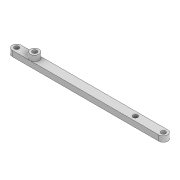
# Autodesk Inventor part: Part_5
Saved by Autodesk Inventor 2022 (Build 260153000, 153)
## iProperties
Created: 2022-04-21
Part Number: Part_5
Material: Generic
Document SubType Name: Modeling
Designer: dell
Density: 1 g/cm^3
Appearance: Default
Author: dell
Autodesk Inventor part; units mm, degrees
ref_plane "YZ Plane" through (0, 0, 0) normal (1, 0, 0) x (0, 1, 0)
ref_plane "XZ Plane" through (0, 0, 0) normal (0, 1, 0) x (-1, 0, 0)
ref_plane "XY Plane" through (0, 0, 0) normal (0, 0, 1) x (1, 0, 0)
sketch "Sketch1" plane through (0, 0, 0) normal (0, 1, 0) x (-1, 0, 0)
  line L0 (0, 0) -> (-132.537, 0) construction
  line L1 (0, 4) -> (-132.537, 4)
  line L2 (-132.537, -4) -> (0, -4)
  arc A0 (0, -4) -> (0, 4) centre (0, 0) ccw
  arc A1 (-132.537, 4) -> (-132.537, -4) centre (-132.537, 0) ccw
  circle A2 centre (0, 0) radius 2.1
  circle A3 centre (-16.286, 0) radius 2.1
  circle A4 centre (-132.537, 0) radius 2.1
  circle A5 centre (-107.252, 0) radius 2.1
  point P0 (-66.2685, 0)
  point P1 (-52.7225, 0)
  dimension "d0" = 132.537
  dimension "d1" = 8
  dimension "d2" = 4.2
  dimension "d8" = 4.2
  dimension "d9" = 16.286
  dimension "d10" = 4.2
  dimension "d28" = 4.2
  dimension "d29" = 107.252
  constraints: 8 end point, 6 centre point, 4 point on circle, 4 tangent, 2 coincident, 2 point on line, 1 horizontal, 1 midpoint, 1 parallel
  measures "d0" distance of L0.end L0.start
  measures "d1" distance between parallel lines of L1 L2
  measures "d2" diameter of A2
  measures "d8" diameter of A3
  measures "d9" distance of L0.start A3.centre
  measures "d10" diameter of A4
  measures "d28" diameter of A5
  measures "d29" distance of L0.start A5.centre
extrude "Extrusion1" add sketch "Sketch1" along normal blind 5
sketch "Sketch4" plane through (0, 5, 0) normal (0, 1, 0) x (1, 0, 0)
  arc A0 (132.537, -4) -> (132.537, 4) centre (132.537, 0) ccw projected
  line L0 (132.537, 4) -> (0, 4) projected
  arc A1 (0, 4) -> (0, -4) centre (0, 0) ccw projected
  line L1 (0, -4) -> (132.537, -4) projected
  circle A2 centre (16.286, 0) radius 2.1 projected
  circle A3 centre (107.252, 0) radius 2.1 projected
  circle A4 centre (132.537, 0) radius 2.1 projected
  circle A5 centre (0, 0) radius 2.1 projected
  circle A6 centre (16.286, 0) radius 4
  dimension "d30" = 8
  constraints: 1 centre point, 1 coincident
  measures "d30" diameter of A6
extrude "Extrusion7" add sketch "Sketch4" along normal blind 5 contours A6
body "Solid1"
